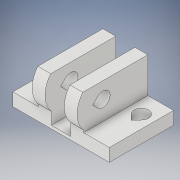
# Autodesk Inventor part: Y-axis Belt Return
Saved by Autodesk Inventor 2018 (Build 220112000, 112)
## iProperties
Created: 2013-10-27
Part Number: Y-axis Belt Return
Material: ASA Plastic
Document SubType Name: Modeling
Designer: Gabriel Smolnycki
Mass: 4.07913 g
Surface Area: 28.7974 cm^2
Volume: 3.81227 cm^3
Density: 1.07 g/cm^3
Appearance: Smooth - White ASA
Sending System: SolidWorks 2017
Last Author: Gabriel Smolnycki
Last Saved: 2017-09-14
Author: Gabriel Smolnycki
Autodesk Inventor part; units mm, degrees
ref_plane "XZ Plane" through (0, 0, 0) normal (0, 1, 0) x (-1, 0, 0)
ref_plane "Work Plane1" through (-15, 0, 0) normal (1, 0, 0) x (0, 1, 0)
sketch "Sketch1" plane through (-15, 0, 0) normal (1, 0, 0) x (0, 1, 0)
  line L0 (0, 20) -> (0, 0)
  arc A0 (15, 20.245) -> (4.7085, 20) centre (10, 14) ccw
  line L1 (15, 0) -> (15, 20.245)
  line L2 (15, 0) -> (0, 0)
  line L3 (4.7085, 20) -> (0, 20)
  constraints: 8 end point, 2 horizontal, 2 point on circle, 2 vertical, 1 centre point
extrude "Extrusion8" add sketch "Sketch1" along normal blind 30
sketch "Sketch2" plane through (15, 0, 0) normal (1, 0, 0) x (0, 0, -1)
  line L0 (-20.245, 15) -> (0, 15)
  line L1 (-20, 4) -> (-20, 4.7085)
  line L2 (0, 4) -> (0, 15)
  arc A0 (-20.245, 15) -> (-20, 4.7085) centre (-14, 10) ccw
  line L3 (-20, 4) -> (0, 4)
  constraints: 8 end point, 2 horizontal, 2 point on circle, 2 vertical, 1 centre point
extrude "Extrusion7" cut sketch "Sketch2" against normal blind 8
sketch "Sketch3" plane through (-15, 0, 0) normal (1, 0, 0) x (0, 1, 0)
  line L0 (4.7085, 20) -> (4, 20)
  line L1 (15, 20.245) -> (15, 0)
  line L2 (4, 20) -> (4, 0)
  arc A0 (15, 20.245) -> (4.7085, 20) centre (10, 14) ccw
  line L3 (15, 0) -> (4, 0)
  constraints: 8 end point, 2 horizontal, 2 point on circle, 2 vertical, 1 centre point
extrude "Extrusion6" cut sketch "Sketch3" along normal blind 8
ref_plane "Work Plane2" through (-3, 0, 0) normal (1, 0, 0) x (0, 1, 0)
sketch "Sketch4" plane through (-3, 0, 0) normal (1, 0, 0) x (0, 1, 0)
  arc A0 (15, 20.245) -> (4.7085, 20) centre (10, 14) ccw
  arc A1 (1, 14) -> (4, 7.2918) centre (10, 14) ccw
  line L0 (15, 20.245) -> (15, 0)
  line L1 (4.7085, 20) -> (1, 20)
  line L2 (4, 7.2918) -> (4, 0)
  line L3 (1, 20) -> (1, 14)
  line L4 (15, 0) -> (4, 0)
  constraints: 10 end point, 4 point on circle, 3 vertical, 2 centre point, 2 horizontal
extrude "Extrusion5" cut sketch "Sketch4" along normal blind 6
sketch "Sketch5" plane through (-3, 4, 7.2918) normal (0, 1, 0) x (1, 0, 0)
  arc A0 (-6.409, -0.2992) -> (-9.591, -0.2992) centre (-8, 1.2918) ccw
  line L0 (-8, -1.8902) -> (-6.409, -0.2992)
  line L1 (-9.591, -0.2992) -> (-8, -1.8902)
  constraints: 4 end point, 2 perpendicular, 2 point on circle, 1 centre point
extrude "Extrusion4" cut sketch "Sketch5" against normal blind 4
sketch "Sketch6" plane through (0, 0, 0) normal (0, 1, 0) x (-1, 0, 0)
  line L0 (-9.409, 7.591) -> (-11, 9.182)
  arc A0 (-12.591, 7.591) -> (-9.409, 7.591) centre (-11, 6) ccw
  line L1 (-11, 9.182) -> (-12.591, 7.591)
  constraints: 4 end point, 2 perpendicular, 2 point on circle, 1 centre point
extrude "Extrusion3" cut sketch "Sketch6" along normal blind 4
sketch "Sketch7" plane through (7, 0, 0) normal (1, 0, 0) x (0, 0, -1)
  arc A0 (-15.591, 8.409) -> (-15.591, 11.591) centre (-14, 10) ccw
  line L0 (-17.182, 10) -> (-15.591, 8.409)
  line L1 (-15.591, 11.591) -> (-17.182, 10)
  constraints: 4 end point, 2 perpendicular, 2 point on circle, 1 centre point
extrude "Extrusion2" cut sketch "Sketch7" against normal blind 4
sketch "Sketch8" plane through (-3, 0, 0) normal (1, 0, 0) x (0, 1, 0)
  arc A0 (8.409, 15.591) -> (11.591, 15.591) centre (10, 14) ccw
  line L0 (8.409, 15.591) -> (10, 17.182)
  line L1 (10, 17.182) -> (11.591, 15.591)
  constraints: 4 end point, 2 perpendicular, 2 point on circle, 1 centre point
extrude "Extrusion1" cut sketch "Sketch8" against normal blind 4 draft 0
body "Solid3"
